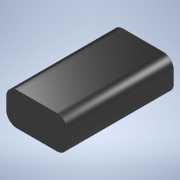
# Autodesk Inventor part: USB C Plug
Saved by Autodesk Inventor 2021 (Build 250183000, 183)
## iProperties
Created: 2024-02-01
Part Number: USB C Plug
Material: Generic
Document SubType Name: Modeling
Designer: maxsm
Density: 1 g/cm^3
Appearance: Default
Author: maxsm
Autodesk Inventor part; units mm, degrees
ref_plane "YZ Plane" through (0, 0, 0) normal (1, 0, 0) x (0, 1, 0)
ref_plane "XZ Plane" through (0, 0, 0) normal (0, 1, 0) x (-1, 0, 0)
ref_plane "XY Plane" through (0, 0, 0) normal (0, 0, 1) x (1, 0, 0)
sketch "Sketch1" plane through (0, 0, 0) normal (0, 0, 1) x (1, 0, 0)
  line L0 (-5.75, 3.1) -> (5.75, 3.1)
  line L1 (5.75, 3.1) -> (5.75, -3.1)
  line L2 (5.75, -3.1) -> (-5.75, -3.1)
  line L3 (-5.75, -3.1) -> (-5.75, 3.1)
  line L4 (-5.75, 3.1) -> (5.75, -3.1) construction
  line L5 (5.75, 3.1) -> (-5.75, -3.1) construction
  point P0 (0, 0)
  dimension "d0" = 11.5
  dimension "d1" = 6.2
  constraints: 12 end point, 2 midpoint, 2 parallel, 1 horizontal, 1 perpendicular
  measures "d0" distance of L1.end L2.end
  measures "d1" distance of L0.end L1.end
extrude "Extrusion1" add sketch "Sketch1" along normal blind 20
fillet "Fillet1" radius 2 4 edges at (5.75, 3.1, 10) (-5.75, 3.1, 10) (-5.75, -3.1, 10) (5.75, -3.1, 10)
body "Solid1"
